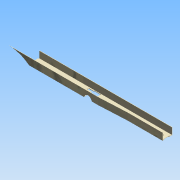
# Autodesk Inventor part: 载板下弹片左
Saved by Autodesk Inventor 2015 (Build 190159000, 159)
## iProperties
Created: 2017-05-16
Part Number: 载板下弹片左
Material: 常规
Document SubType Name: Modeling
Designer: Administrator
Density: 1 g/cm^3
Appearance: 镍
Author: Administrator
Autodesk Inventor part; units mm, degrees
ref_plane "YZ Plane" through (0, 0, 0) normal (1, 0, 0) x (0, 1, 0)
ref_plane "XZ Plane" through (0, 0, 0) normal (0, 1, 0) x (-1, 0, 0)
ref_plane "XY Plane" through (0, 0, 0) normal (0, 0, 1) x (1, 0, 0)
sketch "草图1" plane through (0, 0, 0) normal (0, 0, 1) x (1, 0, 0)
  line L0 (-950, 40) -> (0, 40)
  line L1 (0, 40) -> (0, -40)
  line L2 (0, -40) -> (-950, -40)
  line L3 (-950, -40) -> (-950, 40)
  line L4 (0, -30) -> (-250, -30)
  line L5 (-250, -30) -> (-450, -40)
  point P0 (0, 0)
  point P1 (0, 0)
  dimension "d0" = 950
  dimension "d1" = 80
  dimension "d2" = 250
  dimension "d3" = 200
  dimension "d4" = 10
  constraints: 12 end point, 2 horizontal, 2 parallel, 2 point on line, 1 coincident, 1 midpoint, 1 perpendicular
  measures "d0" distance of L0.start L0.end
  measures "d1" distance of L2.end L0.start
  measures "d2" distance of L4.start L4.end
  measures "d3" horizontal distance of L4.end L5.end
  measures "d4" distance between parallel lines of L2 L4
extrude "拉伸1" add sketch "草图1" along normal blind 50 contours L0 L1 L4 L5 L2 L3
sketch "草图2" plane through (0, -30, 0) normal (1, 0, 0) x (0, 0, -1)
  line L0 (0, 70) -> (0, -10) projected
  line L1 (0, 45) -> (-5, 50)
  line L2 (-5, 50) -> (-5, 10)
  line L3 (-5, 10) -> (0, 15)
  line L4 (0, 45) -> (0, 15)
  point P0 (0, 30)
  dimension "d7" = 40
  dimension "d8" = 20
  dimension "d9" = 135
  dimension "d10" = 5
  constraints: 8 end point, 2 point on line, 1 collinear, 1 parallel, 1 perpendicular
  measures "d7" distance of L1.end L2.end
  measures "d8" vertical distance of point (0, 30) L1.end
  measures "d9" angle of L0 L1
  measures "d10" distance between parallel lines of L0 L2
extrude "拉伸2" cut sketch "草图2" against normal blind 950
shell "抽壳1" thickness 3 removed faces 3 at (-400, 16.6667, 50) at (0, 10, 35) at (-950, -6.6667, 35)
sketch "草图3" plane through (-950, 27.2426, 8) normal (0, 0, 1) x (1, 0, 0)
  circle A0 centre (925, -27.2426) radius 2.5
  line L0 (950, 12.7574) -> (0, 12.7574) projected
  point P0 (950, -27.2426)
  dimension "d14" = 5
  dimension "d15" = 25
  dimension "d16" = 40
  constraints: 1 centre point
  measures "d14" diameter of A0
  measures "d15" distance of point (950, -27.243) A0.centre
  measures "d16" distance from line of L0 A0.centre
extrude "拉伸3" cut sketch "草图3" against normal through all
pattern_linear "矩形阵列1" count 10 spacing 100 along (-1, 0, 0) of "拉伸3"
sketch "草图4" plane through (-950, -40, 0) normal (0, -1, 0) x (1, 0, 0)
  line L0 (0, 0) -> (500, 0) projected
  arc A0 (450, 0) -> (400, 0) centre (425, 0) ccw
  line L1 (403.3494, 12.5) -> (396.1325, 0)
  line L2 (446.6506, 12.5) -> (453.8675, 0)
  line L3 (396.1325, 0) -> (453.8675, 0)
  point P0 (950, 0)
  dimension "d22" = 525
  dimension "d23" = 25
  dimension "d25" = 120
  constraints: 6 end point, 5 point on line, 4 point on circle, 2 tangent, 1 centre point, 1 equal length, 1 horizontal
  measures "d22" distance of point (950, 0) A0.centre
  measures "d23" radius of A0
  measures "d25" angle of L0 L2
extrude "拉伸4" cut sketch "草图4" against normal blind 73
sketch "草图5" plane through (-950, -40, 50) normal (0, -1, 0) x (1, 0, 0)
  line L0 (0, 0) -> (0, -50)
  line L1 (0, 0) -> (-150, 0)
  arc A0 (0, -50) -> (-150, 0) centre (-150, -250) ccw
  line L2 (0, 0) -> (500, 0) projected
  line L3 (0, -50) -> (0, 0) projected
  point P0 (950, -50)
  dimension "d28" = 150
  constraints: 4 end point, 2 collinear, 2 point on circle, 1 centre point, 1 horizontal, 1 tangent, 1 vertical
  measures "d28" distance of L0.start L1.end
extrude "拉伸5" add sketch "草图5" against normal blind 3
fillet "圆角1" radius 3 1 edges at (-1020.9431, -40, 37.1708)
sketch "草图6" plane through (0, 0, 0) normal (0, 0, -1) x (-1, 0, 0)
  line L0 (585.8675, 29) -> (553.8675, 29)
  line L1 (553.8675, 29) -> (553.8675, 12)
  line L2 (553.8675, 12) -> (585.8675, 12)
  line L3 (585.8675, 12) -> (585.8675, 29)
  line L4 (553.8675, 33) -> (553.8675, 15) projected
  line L5 (0, 40) -> (950, 40) projected
  line L6 (553.8675, 12) -> (549.2487, 12)
  line L7 (549.2487, 12) -> (549.2487, 29)
  line L8 (549.2487, 29) -> (553.8675, 29)
  line L9 (553.8675, 29) -> (553.8675, 12)
  line L10 (549.2487, -27.2426) -> (549.2487, 27.2426) projected
  point P0 (0, 0)
  dimension "d32" = 17
  dimension "d33" = 32
  dimension "d34" = 11
  constraints: 16 end point, 4 parallel, 3 collinear, 2 horizontal, 2 perpendicular
  measures "d32" distance of L2.end L0.start
  measures "d33" distance of L0.start L0.end
  measures "d34" distance between parallel lines of L5 L0
extrude "拉伸6" cut sketch "草图6" against normal through all
equation "\"d17\" = d15"
